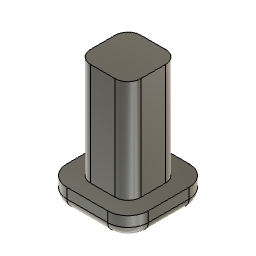
Button v2 (Autodesk Fusion 360 design; units mm, degrees)
Autodesk Fusion 360 part; units mm, degrees
sketch "Base" plane through (0, 0, 0) normal (0, 0, 1) x (1, 0, 0)
  line L0 (3, 0) -> (9, 0)
  line L1 (12, 3) -> (12, 9)
  line L2 (9, 12) -> (3, 12)
  line L3 (0, 9) -> (0, 3)
  arc A0 (3, 12) -> (0, 9) centre (3, 9) ccw
  arc A1 (12, 9) -> (9, 12) centre (9, 9) ccw
  arc A2 (9, 0) -> (12, 3) centre (9, 3) ccw
  arc A3 (0, 3) -> (3, 0) centre (3, 3) ccw
  point P0 (12, 0)
  point P1 (0, 12)
  dimension "d1" = 12
  dimension "d2" = 12
  dimension "d3" = 3
  constraint horizontal L0
  constraint vertical L1
  constraint horizontal L2
  constraint vertical L3
  constraint coincident P1 L2
  constraint coincident P1 L3
  constraint tangent L2 A0
  constraint tangent L3 A0
  constraint tangent L1 A1
  constraint tangent L2 A1
  constraint equal A0 A1
  constraint coincident P0 L0
  constraint coincident P0 L1
  constraint tangent L0 A2
  constraint tangent L1 A2
  constraint equal A0 A2
  constraint coincident origin L0
  constraint coincident origin L3
  constraint tangent L0 A3
  constraint tangent L3 A3
  constraint equal A0 A3
  measures "d1" distance of origin P0
  measures "d2" distance of origin P1
  measures "d3" radius of A0
sketch "Sketch2" plane through (0, 0, 3) normal (0, 0, 1) x (-1, 0, 0)
  arc A0 (0, -3) -> (-3, 0) centre (-3, -3) ccw
  arc A1 (-3, -12) -> (0, -9) centre (-3, -9) ccw
  line L0 (-4.18, -2.28) -> (-7.82, -2.28)
  line L1 (-9.72, -4.18) -> (-9.72, -7.82)
  line L2 (-7.82, -9.72) -> (-4.18, -9.72)
  line L3 (-2.28, -7.82) -> (-2.28, -4.18)
  arc A2 (-4.18, -9.72) -> (-2.28, -7.82) centre (-4.18, -7.82) ccw
  arc A3 (-9.72, -7.82) -> (-7.82, -9.72) centre (-7.82, -7.82) ccw
  arc A4 (-7.82, -2.28) -> (-9.72, -4.18) centre (-7.82, -4.18) ccw
  arc A5 (-2.28, -4.18) -> (-4.18, -2.28) centre (-4.18, -4.18) ccw
  point P0 (-2.28, -2.28)
  point P1 (-9.72, -2.28)
  point P2 (-2.28, -9.72)
  dimension "d18" = 7.44
  dimension "d19" = 7.44
  dimension "d20" = 1.9
  constraint horizontal L0
  constraint vertical L1
  constraint horizontal L2
  constraint vertical L3
  constraint coincident P2 L2
  constraint coincident P2 L3
  constraint tangent L2 A2
  constraint tangent L3 A2
  constraint tangent L1 A3
  constraint tangent L2 A3
  constraint equal A2 A3
  constraint coincident P1 L0
  constraint coincident P1 L1
  constraint tangent L0 A4
  constraint tangent L1 A4
  constraint equal A2 A4
  constraint coincident P0 L0
  constraint coincident P0 L3
  constraint tangent L0 A5
  constraint tangent L3 A5
  constraint equal A2 A5
  measures "d18" distance of P0 P1
  measures "d19" distance of P0 P2
  measures "d20" radius of A2
extrude "Extrude3" add sketch "Base" along normal blind 3
extrude "Extrude4" add sketch "Sketch2" along normal blind 15.143
fillet "Fillet2" radius 1.5 8 edges at (12, 6, 0) (11.1213, 11.1213, 0) (6, 12, 0) (0.8787, 11.1213, 0) (0, 6, 0) (0.8787, 0.8787, 0) (6, 0, 0) (11.1213, 0.8787, 0)
